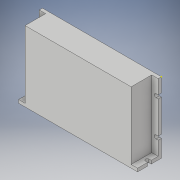
# Autodesk Inventor part: Complete Driver
Saved by Autodesk Inventor 2019 (Build 230136000, 136)
## iProperties
Created: 2020-11-16
Part Number: Complete Driver
Material: Generic
Document SubType Name: Modeling
Designer: Brendan
Density: 1 g/cm^3
Appearance: Default
Author: Brendan
Autodesk Inventor part; units mm, degrees
ref_plane "YZ Plane" through (0, 0, 0) normal (1, 0, 0) x (0, 1, 0)
ref_plane "XZ Plane" through (0, 0, 0) normal (0, 1, 0) x (-1, 0, 0)
ref_plane "XY Plane" through (0, 0, 0) normal (0, 0, 1) x (1, 0, 0)
sketch "Sketch1" plane through (0, 0, 0) normal (0, 0, 1) x (1, 0, 0)
  point P0 (0, 0)
sketch "Sketch2" plane through (0, 0, 0) normal (0, 0, 1) x (1, 0, 0)
  line L0 (0, 0) -> (-166, 0)
  line L1 (-166, -98.3) -> (0, -98.3)
  line L2 (0, 0) -> (-163, 0)
  line L3 (0, -19.5) -> (0, 0)
  line L4 (-3, 0) -> (0, 0)
  line L5 (0, 0) -> (0, -19.5)
  line L6 (-166, -19.5) -> (-163, -19.5)
  line L7 (-166, -24.5) -> (-163, -24.5)
  line L8 (-166, -98.3) -> (-3, -98.3)
  line L9 (-166, -74.3) -> (-166, -98.3)
  line L10 (-163, -98.3) -> (-166, -98.3)
  line L11 (-166, -98.3) -> (-166, -74.3)
  line L12 (-163, -69.3) -> (-166, -69.3)
  line L13 (-166, -74.3) -> (-163, -74.3)
  arc A0 (-163, -74.3) -> (-163, -69.3) centre (-163, -71.8) ccw
  line L14 (-166, -74.3) -> (-166, -98.3)
  line L15 (-166, 0) -> (-166, -19.5)
  line L16 (-166, -24.5) -> (-166, -69.3)
  line L17 (0, -69.3) -> (-3, -69.3)
  line L18 (-3, -69.3) -> (0, -69.3)
  line L19 (0, -74.3) -> (-3, -74.3)
  arc A1 (-3, -69.3) -> (-3, -74.3) centre (-3, -71.8) ccw
  arc A2 (-163.2703, -24.5) -> (-163.2703, -19.5) centre (-163.2703, -22) ccw
  line L20 (0, -98.3) -> (0, -74.3)
  line L21 (-163.2703, -19.5) -> (-163, -19.5)
  line L22 (-163, -24.5) -> (-163.2703, -24.5)
  line L23 (0, -19.5) -> (-3, -19.5)
  line L24 (-3, -24.5) -> (0, -24.5)
  arc A3 (-3, -19.5) -> (-3, -24.5) centre (-3, -22) ccw
  line L25 (-3.2703, -19.5) -> (-3.2703, -19.5147)
  line L26 (-3.2703, -24.4853) -> (-3.2703, -24.5)
  line L27 (0, -69.3) -> (0, -24.5)
  line L28 (0, -19.5) -> (0, 0)
  dimension "d19" = 160
  dimension "d21" = 49.8
  constraints: 58 end point, 13 parallel, 10 point on circle, 6 horizontal, 5 perpendicular, 4 centre point, 2 point on line, 1 tangent
  measures "d19" distance of L26.end L22.end
  measures "d21" distance of A1.centre A3.centre
extrude "Extrusion1" add sketch "Sketch2" along normal blind 33.2
sketch "Sketch3" plane through (0, 0, 33.2) normal (0, 0, 1) x (1, 0, 0)
  line L0 (-9, 0) -> (-9, -93.8)
  line L1 (-166, -93.8) -> (-166, 0)
  line L2 (-157, 0) -> (-157, -93.8)
  line L3 (-9, -93.8) -> (-9, 0)
  line L4 (-9, -93.8) -> (0, -93.8)
  line L5 (0, -93.8) -> (0, 0)
  line L6 (0, 0) -> (-9, 0)
  line L7 (-9, 0) -> (-9, -93.8)
  line L8 (-166, 0) -> (-166, -19.5) projected
  line L9 (-166, 0) -> (-157, 0)
  line L10 (-157, 0) -> (-157, -93.8)
  line L11 (-157, -93.8) -> (-166, -93.8)
  line L12 (-166, -93.8) -> (-166, 0)
  dimension "d24" = 157
  dimension "d25" = 93.8
  dimension "d26" = 148
  constraints: 24 end point, 6 parallel, 2 horizontal, 2 perpendicular
  measures "d24" distance of L0.end L1.start
  measures "d25" distance of L0.start L0.end
  measures "d26" distance of L3.start L2.end
extrude "Extrusion2" cut sketch "Sketch3" against normal blind 28.7
sketch "Sketch4" plane through (-166, -98.3, 0) normal (0, -1, 0) x (1, 0, 0)
  line L0 (166, 33.2) -> (163, 33.2)
  line L1 (166, 19.3) -> (166, 33.2)
  line L2 (166, 0) -> (166, 33.2) projected
  line L3 (166, 19.3) -> (163, 19.3)
  line L4 (166, 14.3) -> (163, 14.3)
  arc A0 (163, 19.3) -> (163, 14.3) centre (163, 16.8) ccw
  line L5 (0, 33.2) -> (166, 33.2) projected
  line L6 (0, 33.2) -> (3, 33.2)
  line L7 (0, 14.3) -> (3, 14.3)
  line L8 (0, 19.3) -> (3, 19.3)
  arc A1 (3, 14.3) -> (3, 19.3) centre (3, 16.8) ccw
  line L9 (0, 19.3) -> (0, 14.3)
  line L10 (0, 0) -> (0, 33.2) projected
  constraints: 16 end point, 4 point on circle, 2 centre point, 2 horizontal, 2 point on line, 1 collinear
extrude "Extrusion3" cut sketch "Sketch4" against normal blind 28.7
body "Solid1"
